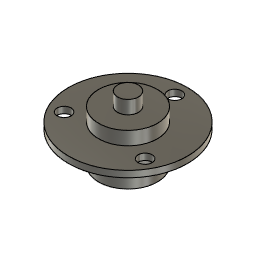
RAD-AlecBearing with Warp Plate Key (Autodesk Fusion 360 archive; units mm, degrees)
design "Slip Ring SNM022A-06"
Autodesk Fusion 360 part; units mm, degrees
sketch "Sketch1" plane through (0, 0, 0) normal (0, 0, 1) x (1, 0, 0)
  circle A0 centre (0, 0) radius 22.25
  circle A1 centre (0, 0) radius 17.5
  circle A2 centre (0, 0) radius 11
  line L0 (0, 0) -> (0, 30)
  circle A3 centre (0, 17.5) radius 2.6
  circle A4 centre (-15.1554, -8.75) radius 2.6
  circle A5 centre (15.1554, -8.75) radius 2.6
  circle A6 centre (0, 0) radius 3.9
  dimension "d1" = 44.5
  dimension "d2" = 35
  dimension "d3" = 22
  dimension "d4" = 5.2
  dimension "d5" = 5.2
  dimension "d6" = 5.2
  dimension "d7" = 7.8
  constraint coincident A0.centre A1.centre
  constraint concentric A0 A1
  constraint concentric A1 A2
  constraint vertical L0
  constraint coincident A1 A3.centre
  constraint coincident L0 A3.centre
  measures "d1" diameter of A0
  measures "d2" diameter of A1
  measures "d3" diameter of A2
  measures "d4" diameter of A3
  measures "d5" diameter of A4
  measures "d6" diameter of A5
  measures "d7" diameter of A6
extrude "Extrude1" add sketch "Sketch1" against normal blind 2.4 contours A0 | A1 A3 A4 A5 | A2 | A6
extrude "Extrude2" add sketch "Sketch1" along normal blind 5 and the other way blind 14 contours A2 | A6
extrude "Extrude3" add sketch "Sketch1" along normal blind 10 contours A6
